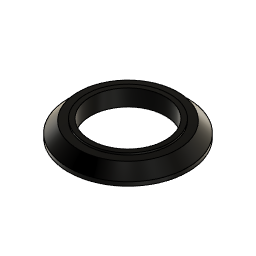
A-1122 nut washer (Autodesk Fusion 360 design; units mm, degrees)
Autodesk Fusion 360 part; units mm, degrees
sketch "Sketch2" plane through (0, 0, 0) normal (0, 1, 0) x (1, 0, 0)
  line L0 (0, -5.5) -> (0, 3.2)
  line L1 (0, 0) -> (4.9, 0) construction
  line L2 (4.9, 0) -> (4.9, -2.15)
  line L3 (4.9, 0) -> (7.8, 0)
  line L4 (7.8, 0) -> (7.8, -0.5)
  line L5 (4.9, -2.15) -> (5.5, -2.15)
  line L6 (5.5, -2.15) -> (5.5, -1.9)
  line L7 (5.5, -1.9) -> (6.5, -1.9)
  line L8 (6.5, -1.9) -> (7.8, -0.5)
  dimension "d3" = 4.9
  dimension "d4" = 2.15
  dimension "d5" = 2.9
  dimension "d6" = 0.5
  dimension "d7" = 0.6
  dimension "d8" = 1.9
  dimension "d9" = 1.6
  constraint vertical L0
  constraint coincident L1.start origin
  constraint perpendicular L0 L1
  constraint perpendicular L1 L2
  constraint perpendicular L2 L3
  constraint perpendicular L3 L4
  constraint perpendicular L2 L5
  constraint perpendicular L5 L6
  constraint perpendicular L6 L7
  measures "d3" distance of L1.start L1.end
  measures "d4" distance of L1.end L2.end
  measures "d5" distance of L1.end L3.end
  measures "d6" distance of L3.end L4.end
  measures "d7" distance of L2.end L5.end
  measures "d8" distance of L3 L7
  measures "d9" distance of L2 L7.end
revolve "Revolve1" add sketch "Sketch2" angle 360 about axis through (0, 0, 5.5) along (0, 0, -1)
equation "d3 = ( 9.8 / 2 ) * 1 mm"
equation "d5 = ( 15.6 / 2 ) * 1 mm - 4.9 mm"
